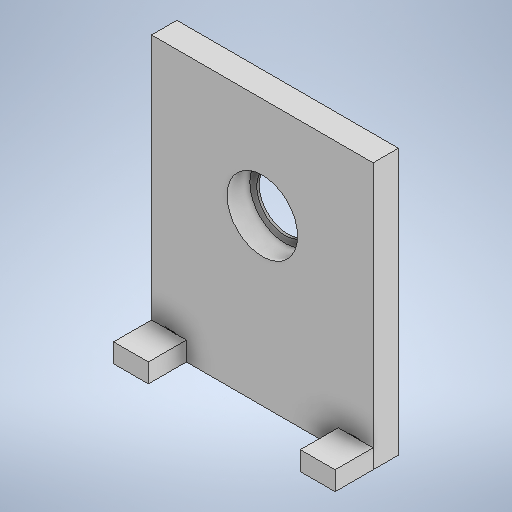
# Autodesk Inventor part: Turm_Idler
Saved by Autodesk Inventor 2025 (Build 290162000, 162)
## iProperties
Created: 2026-07-10
Part Number: Turm_Idler
Material: Generisch
Document SubType Name: Modeling
Designer: wavid
Mass: 45.552 g
Surface Area: 153.688 cm^2
Volume: 45.552 cm^3
Density: 1 g/cm^3
Appearance: Vorgabe
Author: wavid
Autodesk Inventor part; units mm, degrees
ref_plane "YZ Plane" through (0, 0, 0) normal (1, 0, 0) x (0, 1, 0)
ref_plane "XZ Plane" through (0, 0, 0) normal (0, 1, 0) x (-1, 0, 0)
ref_plane "XY Plane" through (0, 0, 0) normal (0, 0, 1) x (1, 0, 0)
sketch "Skizze1" plane through (0, 0, 0) normal (0, 0, 1) x (1, 0, 0)
  line L0 (-35, 0) -> (35, 0)
  line L1 (35, 0) -> (35, 8)
  line L2 (35, 8) -> (-35, 8)
  line L3 (-35, 8) -> (-35, 0)
  constraints: 8 end point, 2 parallel, 1 horizontal, 1 perpendicular
extrude "Extrusion1" add sketch "Skizze1" along normal blind 84
sketch "Skizze2" plane through (0, 0, 0) normal (0, 0, 1) x (1, 0, 0)
  line L0 (-35, -12) -> (-24, -12)
  line L1 (-24, -12) -> (-24, 0)
  line L2 (-24, 0) -> (-35, 0)
  line L3 (-35, 0) -> (-35, -12)
  constraints: 8 end point, 2 parallel, 1 horizontal, 1 perpendicular
extrude "Extrusion2" add sketch "Skizze2" along normal blind 6 separate body
sketch "Skizze3" plane through (0, 0, 0) normal (0, 0, 1) x (1, 0, 0)
  line L0 (24, -12) -> (35, -12)
  line L1 (35, -12) -> (35, 0)
  line L2 (35, 0) -> (24, 0)
  line L3 (24, 0) -> (24, -12)
  constraints: 8 end point, 2 parallel, 1 horizontal, 1 perpendicular
extrude "Extrusion3" add sketch "Skizze3" along normal blind 6 separate body
sketch "Skizze4" plane through (0, 0, 0) normal (0, 0, 1) x (1, 0, 0)
  circle A0 centre (-29, 0) radius 1.7
  constraints: 1 centre point
extrude "Extrusion4" cut sketch "Skizze4" along normal blind 6.2 bodies 1
sketch "Skizze5" plane through (0, 0, 0) normal (0, 0, 1) x (1, 0, 0)
  circle A0 centre (29, 0) radius 1.7
  constraints: 1 centre point
extrude "Extrusion5" cut sketch "Skizze5" along normal blind 6.2 bodies 1
sketch "Skizze6" plane through (0, 0, 0) normal (0, 1, 0) x (-1, 0, 0)
  circle A0 centre (0, 52) radius 11.15
  constraints: 1 centre point
extrude "Extrusion6" cut sketch "Skizze6" along normal blind 7.2 bodies 1
sketch "Skizze7" plane through (0, 0, 0) normal (0, 1, 0) x (-1, 0, 0)
  circle A0 centre (0, 52) radius 9
  constraints: 1 centre point
extrude "Extrusion7" cut sketch "Skizze7" along normal blind 8.2 bodies 1
